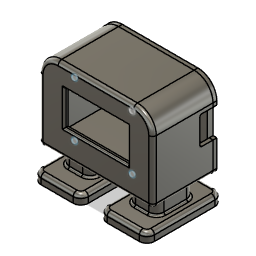
sparky v67 (Autodesk Fusion 360 design; units mm, degrees)
Autodesk Fusion 360 part; units mm, degrees
note: some values were not read from the file. Chosen so that the rebuilt part matches the saved one: which bodies a step acts on; which face or edge a step refers to; which pieces of a blend or face edit are solid.
sketch "Skizze7" plane through (0, 0, 0) normal (0, 1, 0) x (1, 0, 0)
  line L0 (-35, 20) -> (-10, 20)
  line L1 (-10, 20) -> (-10, -20)
  line L2 (-10, -20) -> (-35, -20)
  line L3 (-35, -20) -> (-35, 20)
  line L4 (0, -25) -> (0, 25) construction
  line L5 (35, 20) -> (10, 20)
  line L6 (10, 20) -> (10, -20)
  line L7 (10, -20) -> (35, -20)
  line L8 (35, -20) -> (35, 20)
  dimension "d14" = 25
  dimension "d15" = 40
  constraint horizontal L0
  constraint vertical L1
  constraint horizontal L2
  constraint vertical L3
  constraint parallel L1 L4
  constraint symmetric L0.start L4 L5.start
  constraint symmetric L0.end L4 L5.end
  constraint symmetric L1.end L4 L6.end
  constraint symmetric L2.end L4 L7.end
  measures "d14" distance of L0.start L0.end
  measures "d15" distance of L0.start L2.end
extrude "Extrusion1" add sketch "Skizze7" along normal blind 5 makes body 1 at (-26.6667, 0, -6.6667) makes body 2 at (18.3333, 0, -6.6667)
sketch "Skizze8" plane through (0, 5, 0) normal (0, 1, 0) x (-1, 0, 0)
  line L0 (35, 20) -> (10, 20)
  line L1 (10, 20) -> (10, -20)
  line L2 (10, -20) -> (35, -20)
  line L3 (35, -20) -> (35, 20)
sketch "Skizze9" plane through (0, 5, 0) normal (0, 1, 0) x (-1, 0, 0)
  line L0 (15, -10) -> (27.5, -10)
  line L1 (27.5, -10) -> (27.5, 10)
  line L2 (27.5, 10) -> (15, 10)
  line L3 (15, 10) -> (15, -10)
  line L4 (0, -20) -> (0, 20) construction
  line L5 (-15, -10) -> (-27.5, -10)
  line L6 (-27.5, -10) -> (-27.5, 10)
  line L7 (-27.5, 10) -> (-15, 10)
  line L8 (-15, 10) -> (-15, -10)
  dimension "d18" = 12.5
  dimension "d19" = 20
  constraint horizontal L0
  constraint vertical L1
  constraint horizontal L2
  constraint vertical L3
  constraint perpendicular L0 L4
  constraint symmetric L0.start L4 L5.start
  constraint symmetric L0.end L4 L5.end
  constraint symmetric L1.end L4 L6.end
  constraint symmetric L2.end L4 L7.end
  measures "d18" distance of L0.start L0.end
  measures "d19" distance of L0.start L2.end
extrude "Extrusion2" add sketch "Skizze9" along normal blind 10 bodies 1 2
sketch "Skizze10" plane through (0, 15, 0) normal (0, 1, 0) x (-1, 0, 0)
  line L0 (15, 10) -> (15, -10)
  line L1 (15, -10) -> (27.5, -10)
  line L2 (27.5, -10) -> (27.5, 10)
  line L3 (27.5, 10) -> (15, 10)
  line L4 (-30, -18) -> (30, -18)
  line L5 (30, -18) -> (30, 18)
  line L6 (30, 18) -> (-30, 18)
  line L7 (-30, 18) -> (-30, -18)
  line L8 (-30, -18) -> (30, 18) construction
  line L9 (30, -18) -> (-30, 18) construction
  dimension "d22" = 60
  dimension "d23" = 36
  constraint horizontal L4
  constraint perpendicular L4 L5
  constraint parallel L4 L6
  constraint parallel L5 L7
  constraint coincident L8 origin
  constraint coincident L9 origin
  measures "d22" distance of L5.end L6.end
  measures "d23" distance of L4.end L5.end
extrude "Extrusion3" add sketch "Skizze10" along normal blind 40 contours L0 L1 L2 L3 | L4 L5 L6 L7 bodies 1 2
sketch "Skizze11" plane through (0, 0, -18) normal (0, 0, -1) x (-1, 0, 0)
  line L0 (-30, 15) -> (30, 15)
  line L1 (30, 15) -> (30, 55)
  line L2 (30, 55) -> (-30, 55)
  line L3 (-30, 55) -> (-30, 15)
  line L4 (0, 55) -> (0, 25) construction
  constraint midpoint L2 L4.start
  constraint perpendicular L0 L4
sketch "Skizze12" plane through (0, 0, -18) normal (0, 0, -1) x (1, 0, 0)
ref_plane "Arbeitsebene4" through (0, 35, -14) normal (0, 0, -1) x (-1, 0, 0)
split "Teilen1" by plane through (0, 35, -14) normal (0, 0, -1) bodies 1 makes body 3 at (-26.6667, 5, -18) makes body 4 at (26.6667, 5, -16) makes body 5 at (10, 28.3333, -18)
combine "Kombinieren1" operation add target body 1 tool bodies 3 4
sketch "Skizze13" plane through (0, 0, -14) normal (0, 0, -1) x (-1, 0, 0)
  line L0 (-30, 15) -> (30, 15)
  line L1 (30, 15) -> (30, 55)
  line L2 (30, 55) -> (-30, 55)
  line L3 (-30, 55) -> (-30, 15)
  line L4 (-28, 73) -> (28, 73)
  line L5 (28, 73) -> (28, 17)
  line L6 (28, 17) -> (-28, 17)
  line L7 (-28, 17) -> (-28, 73)
  constraint horizontal L4
  constraint vertical L5
  constraint horizontal L6
  constraint vertical L7
extrude "Extrusion4" cut sketch "Skizze13" against normal blind 30 contours L2 L4 L5 L7 | L2 L5 L6 L7 bodies 1
split "Teilen2" by plane through (0, 15, 0) normal (0, -1, 0) bodies 1 makes body 6 at (26.6667, 0, 6.6667) makes body 7 at (-26.6667, 0, -6.6667)
sketch "Skizze14" plane through (0, 15, 0) normal (0, 1, 0) x (-1, 0, 0)
  line L0 (-15, 10) -> (-27.5, 10)
  line L1 (-27.5, 10) -> (-27.5, -10)
  line L2 (-27.5, -10) -> (-15, -10)
  line L3 (-15, -10) -> (-15, 10)
  circle A0 centre (-21.25, 0.004) radius 2
  line L4 (0, 25) -> (0, -25) construction
  circle A1 centre (21.25, 0.004) radius 2
  dimension "d29" = 4
  constraint vertical L4
  constraint symmetric A0 L4 A1
  measures "d29" diameter of A0
sketch "Skizze16" plane through (0, 55, 0) normal (0, 1, 0) x (-1, 0, 0)
  line L0 (28, 16) -> (28, -14)
  line L1 (28, -14) -> (30, -14)
  line L2 (30, -14) -> (30, 18)
  line L3 (30, 18) -> (-30, 18)
  line L4 (-30, 18) -> (-30, -14)
  line L5 (-30, -14) -> (-28, -14)
  line L6 (-28, -14) -> (-28, 16)
  line L7 (-28, 16) -> (28, 16)
  line L8 (-30, 18) -> (30, 18)
  line L9 (30, 18) -> (30, -14)
  line L10 (30, -14) -> (-30, -14)
  line L11 (-30, -14) -> (-30, 18)
  constraint horizontal L8
  constraint vertical L9
  constraint horizontal L10
  constraint vertical L11
  constraint coincident L1.end L2.start
  constraint coincident L3.end L4.start
extrude "Extrusion6" add sketch "Skizze16" along normal blind 3 contours L0 L1 L2 L3 L4 L5 L6 L7 L8 L9 L10 L11 bodies 1
sketch "Skizze17" plane through (-28, 0, 0) normal (1, 0, 0) x (0, 0, -1)
  line L0 (-16, 58) -> (-16, 17)
  line L1 (-16, 17) -> (14, 17)
  line L2 (14, 17) -> (14, 58)
  line L3 (14, 58) -> (-16, 58)
  line L4 (14, 58) -> (-16, 58)
  line L5 (-16, 58) -> (-16, 56)
  line L6 (-16, 56) -> (14, 56)
  line L7 (14, 56) -> (14, 58)
  constraint horizontal L4
  constraint vertical L5
  constraint horizontal L6
  constraint vertical L7
  constraint coincident L0 L5.end
  constraint coincident L2.end L3.start
extrude "Extrusion7" add sketch "Skizze17" along normal blind 56 contours L0 L2 L3 L4 L5 L6 L7 bodies 1
sketch "Skizze18" plane through (0, 0, 18) normal (0, 0, 1) x (1, 0, 0)
  line L0 (-30, 15) -> (30, 15)
  line L1 (30, 15) -> (30, 58)
  line L2 (30, 58) -> (-30, 58)
  line L3 (-30, 58) -> (-30, 15)
ref_plane "WorkPlane5" through (0, 36.5, 19) normal (0, 0, 1) x (1, 0, 0)
sketch "Sketch19" plane through (0, 0, 19) normal (0, 0, 1) x (1, 0, 0)
  line L0 (-25, 20) -> (25, 20)
  line L1 (25, 20) -> (25, 55)
  line L2 (25, 55) -> (-25, 55)
  line L3 (-25, 55) -> (-25, 20)
  constraint horizontal L0
  constraint vertical L1
  constraint horizontal L2
  constraint vertical L3
sketch "Sketch20" plane through (0, 0, 19) normal (0, 0, 1) x (1, 0, 0)
  line L0 (-17.75, 25) -> (17.75, 25)
  line L1 (17.75, 25) -> (17.75, 48)
  line L2 (17.75, 48) -> (-17.75, 48)
  line L3 (-17.75, 48) -> (-17.75, 25)
  line L4 (-30, 58) -> (-30, 15)
  line L5 (30, 15) -> (30, 58)
  line L6 (30, 58) -> (-30, 58)
  line L7 (-30, 15) -> (30, 15)
  dimension "d37" = 35.5
  dimension "d38" = 23
  dimension "d39" = 12.25
  dimension "d40" = 12.25
  dimension "d41" = 10
  dimension "d42" = 10
  constraint horizontal L0
  constraint vertical L1
  constraint horizontal L2
  constraint vertical L3
  measures "d37" distance of L0.start L0.end
  measures "d38" distance of L0.start L2.end
  measures "d39" distance of L3 L4
  measures "d40" distance of L1 L5
  measures "d41" distance of L2 L6
  measures "d42" distance of L0 L7
extrude "Extrude8" cut sketch "Sketch20" against normal blind 10 contours L0 L1 L2 L3 bodies 1
fillet "Fillet1" radius 8 2 edges at (28, 56, 1) (-28, 56, 1) on bodies 1
fillet "Fillet2" radius 10 2 edges at (-30, 58, 2) (30, 58, 2) on bodies 1
fillet "Fillet3" radius 4 6 edges at (0, 15, 18) (-30, 31.5, 18) (-27.0711, 55.0711, 18) (0, 58, 18) (27.0711, 55.0711, 18) (30, 31.5, 18) on bodies 1
fillet "Fillet4" radius 1 4 edges at (0, 25, 18) (17.75, 36.5, 18) (0, 48, 18) (-17.75, 36.5, 18) on bodies 1
fillet "Fillet5" radius 2 4 edges at (28.8284, 16.1716, 16.8284) (30, 15, 0) (-30, 15, 0) (-28.8284, 16.1716, 16.8284) on bodies 1
fillet "Fillet6" radius 1 2 edges at (-28, 17, 1) (28, 17, 1) on bodies 1
move_body "Move1" bodies 7 to x (1, 0, 0) y (0, 1, 0) z (0, 0, 1) at (-40, 0, 0)
extrude "Extrude9" add 1 faces at (-67.5, 8.3333, -3.3333) along direction (-1, 0, 0) blind 2.5 on bodies 7 bodies 7
delete_body "RemoveBody1" bodies 6
fillet "Fillet7" radius 4 4 edges at (-75, 2.5, 20) (-50, 2.5, 20) (-75, 2.5, -20) (-50, 2.5, -20) on bodies 7
fillet "Fillet8" radius 4 4 edges at (-70, 10, -10) (-70, 10, 10) (-55, 10, -10) (-55, 10, 10) on bodies 7
fillet "Fillet9" radius 2 8 edges at (-73.8284, 5, 18.8284) (-62.5, 5, 20) (-51.1716, 5, 18.8284) (-50, 5, 0) (-51.1716, 5, -18.8284) (-62.5, 5, -20) (-73.8284, 5, -18.8284) (-75, 5, 0) on bodies 7
fillet "Fillet10" radius 1 8 edges at (-56.1716, 5, -8.8284) (-55, 5, 0) (-56.1716, 5, 8.8284) (-62.5, 5, 10) (-68.8284, 5, 8.8284) (-70, 5, 0) (-68.8284, 5, -8.8284) (-62.5, 5, -10) on bodies 7
sketch "Sketch21" plane through (0, 15, 0) normal (0, 1, 0) x (-1, 0, 0)
  arc A0 (59, 10) -> (55, 6) centre (59, 6) ccw
  line L0 (55, 6) -> (55, -6)
  arc A1 (55, -6) -> (59, -10) centre (59, -6) ccw
  line L1 (59, -10) -> (66, -10)
  arc A2 (66, -10) -> (70, -6) centre (66, -6) ccw
  line L2 (70, -6) -> (70, 6)
  arc A3 (70, 6) -> (66, 10) centre (66, 6) ccw
  line L3 (66, 10) -> (59, 10)
  line L4 (57.5, 7.5) -> (67.5, 7.5)
  line L5 (67.5, 7.5) -> (67.5, -7.5)
  line L6 (67.5, -7.5) -> (57.5, -7.5)
  line L7 (57.5, -7.5) -> (57.5, 7.5)
  point P0 (62.5, 0)
  dimension "d67" = 7.5
  dimension "d68" = 10
  constraint horizontal L4
  constraint vertical L5
  constraint horizontal L6
  constraint vertical L7
  measures "d67" distance of L2 P0
  measures "d68" distance of L1 P0
extrude "Extrude10" cut sketch "Sketch21" against normal blind 10 contours L4 L5 L6 L7 bodies 7
fillet "Fillet11" radius 2 1 edges at (-57.5, 10, 7.5) on bodies 7
fillet "Fillet12" radius 2 3 edges at (-67.5, 10, 7.5) (-67.5, 10, -7.5) (-57.5, 10, -7.5) on bodies 7
move_body "Move2" bodies 7 to x (1, 0, 0) y (0, 1, 0) z (0, 0, 1) at (45, 0, 0)
move_body "Move3" bodies 7 to x (1, 0, 0) y (0, 1, 0) z (0, 0, 1) at (0, 0, 1)
copy_body "CopyPasteBodies1" bodies 7 makes body 8
move_body "Move4" bodies 8 to x (1, 0, 0) y (0, 1, 0) z (0, 0, 1) at (35, 0, 0)
sketch "Sketch22" plane through (0, 0, -14) normal (0, 0, -1) x (-1, 0, 0)
  arc A0 (28, 15) -> (30, 17) centre (28, 17) ccw
  line L0 (30, 17) -> (30, 48)
  arc A1 (30, 48) -> (20, 58) centre (20, 48) ccw
  line L1 (20, 58) -> (-20, 58)
  arc A2 (-20, 58) -> (-30, 48) centre (-20, 48) ccw
  line L2 (-30, 48) -> (-30, 17)
  arc A3 (-30, 17) -> (-28, 15) centre (-28, 17) ccw
  line L3 (-28, 15) -> (28, 15)
  arc A4 (27, 17) -> (28, 18) centre (27, 18) ccw
  line L4 (27, 17) -> (-27, 17)
  arc A5 (-28, 18) -> (-27, 17) centre (-27, 18) ccw
  line L5 (-28, 18) -> (-28, 48)
  arc A6 (-20, 56) -> (-28, 48) centre (-20, 48) ccw
  line L6 (-20, 56) -> (20, 56)
  arc A7 (28, 48) -> (20, 56) centre (20, 48) ccw
  line L7 (28, 48) -> (28, 18)
extrude "Extrude11" add sketch "Sketch22" along normal blind 2 separate body makes body 9
delete_body "RemoveBody2" bodies 5
delete_face "DeleteFace1" 1 faces at (27.9989, 17.9524, -14.6667) on bodies 9
delete_face "DeleteFace2" 1 faces at (-27.5, 17.134, -15.3333) on bodies 9
extrude "Extrude12" add 1 faces at (6.6667, 56, -14.6667) along direction (0, -1, 0) blind 40 on bodies 9 bodies 9
extrude "Extrude13" add 1 faces at (22.6667, 17, -14.6667) along direction (0, 1, 0) blind 31 on bodies 9 bodies 9
extrude "Extrude14" add 1 faces at (-25.3333, 17, -14.6667) along direction (0, 1, 0) blind 31 on bodies 9 bodies 9
sketch "Sketch23" plane through (0, 0, -16) normal (0, 0, -1) x (-1, 0, 0)
  arc A0 (-20, 56) -> (-28, 48) centre (-20, 48) ccw
  line L0 (-20, 56) -> (-20, 48)
  line L1 (-20, 48) -> (-28, 48)
  line L2 (-28, 15) -> (28, 15)
  arc A1 (28, 15) -> (30, 17) centre (28, 17) ccw
  line L3 (30, 17) -> (30, 48)
  arc A2 (30, 48) -> (20, 58) centre (20, 48) ccw
  line L4 (20, 58) -> (-20, 58)
  arc A3 (-20, 58) -> (-30, 48) centre (-20, 48) ccw
  line L5 (-30, 48) -> (-30, 17)
  arc A4 (-30, 17) -> (-28, 15) centre (-28, 17) ccw
  line L6 (20, 48) -> (20, 56)
  arc A5 (28, 48) -> (20, 56) centre (20, 48) ccw
  line L7 (28, 48) -> (20, 48)
extrude "Extrude15" add sketch "Sketch23" against normal blind 2 contours A0 L0 L1 bodies 9
sketch "Sketch24" plane through (0, 0, -16) normal (0, 0, -1) x (-1, 0, 0)
  line L0 (-28, 15) -> (28, 15)
  arc A0 (28, 15) -> (30, 17) centre (28, 17) ccw
  line L1 (30, 17) -> (30, 48)
  arc A1 (30, 48) -> (20, 58) centre (20, 48) ccw
  line L2 (20, 58) -> (-20, 58)
  arc A2 (-20, 58) -> (-30, 48) centre (-20, 48) ccw
  line L3 (-30, 48) -> (-30, 17)
  arc A3 (-30, 17) -> (-28, 15) centre (-28, 17) ccw
  line L4 (20, 48) -> (20, 56)
  arc A4 (28, 48) -> (20, 56) centre (20, 48) ccw
  line L5 (28, 48) -> (20, 48)
extrude "Extrude16" add sketch "Sketch24" against normal blind 2 contours L4 A4 L5 bodies 9
delete_face "DeleteFace3" 1 faces at (27.3717, 17.0716, -4) on bodies 1
delete_face "DeleteFace4" 1 faces at (-27.0951, 17.0045, -4) on bodies 1
sketch "Sketch25" plane through (0, 0, 16) normal (0, 0, -1) x (-1, 0, 0)
  line L0 (17.75, 25) -> (-17.75, 25)
  line L1 (-17.75, 25) -> (-17.75, 48)
  line L2 (-17.75, 48) -> (17.75, 48)
  line L3 (17.75, 48) -> (17.75, 25)
  line L4 (28, 17) -> (28, 48)
  arc A0 (28, 48) -> (20, 56) centre (20, 48) ccw
  line L5 (20, 56) -> (-20, 56)
  arc A1 (-20, 56) -> (-28, 48) centre (-20, 48) ccw
  line L6 (-28, 48) -> (-28, 17)
  line L7 (-28, 17) -> (28, 17)
move_body "Move5" bodies 8 7 to x (1, 0, 0) y (0, 1, 0) z (0, 0, 1) at (0, -10, 0)
sketch "Sketch26" plane through (0, 15, 0) normal (0, -1, 0) x (1, 0, 0)
  line L0 (-28, 14) -> (-28, -14)
  line L1 (-28, -14) -> (28, -14)
  line L2 (28, -14) -> (28, 14)
  line L3 (28, 14) -> (-28, 14)
  line L4 (12.5, 6.5) -> (12.5, -4.5)
  arc A0 (12.5, -4.5) -> (14.5, -6.5) centre (14.5, -4.5) ccw
  line L5 (14.5, -6.5) -> (20.5, -6.5)
  arc A1 (20.5, -6.5) -> (22.5, -4.5) centre (20.5, -4.5) ccw
  line L6 (22.5, -4.5) -> (22.5, 6.5)
  arc A2 (22.5, 6.5) -> (20.5, 8.5) centre (20.5, 6.5) ccw
  line L7 (20.5, 8.5) -> (14.5, 8.5)
  arc A3 (14.5, 8.5) -> (12.5, 6.5) centre (14.5, 6.5) ccw
  arc A4 (25, 7) -> (21, 11) centre (21, 7) ccw
  line L8 (25, 7) -> (25, -5)
  arc A5 (21, -9) -> (25, -5) centre (21, -5) ccw
  line L9 (21, -9) -> (14, -9)
  arc A6 (10, -5) -> (14, -9) centre (14, -5) ccw
  line L10 (10, -5) -> (10, 7)
  arc A7 (14, 11) -> (10, 7) centre (14, 7) ccw
  line L11 (14, 11) -> (21, 11)
  line L12 (-22.5, 6.5) -> (-22.5, -4.5)
  arc A8 (-22.5, -4.5) -> (-20.5, -6.5) centre (-20.5, -4.5) ccw
  line L13 (-20.5, -6.5) -> (-14.5, -6.5)
  arc A9 (-14.5, -6.5) -> (-12.5, -4.5) centre (-14.5, -4.5) ccw
  line L14 (-12.5, -4.5) -> (-12.5, 6.5)
  arc A10 (-12.5, 6.5) -> (-14.5, 8.5) centre (-14.5, 6.5) ccw
  line L15 (-14.5, 8.5) -> (-20.5, 8.5)
  arc A11 (-20.5, 8.5) -> (-22.5, 6.5) centre (-20.5, 6.5) ccw
  arc A12 (-10, 7) -> (-14, 11) centre (-14, 7) ccw
  line L16 (-10, 7) -> (-10, -5)
  arc A13 (-14, -9) -> (-10, -5) centre (-14, -5) ccw
  line L17 (-14, -9) -> (-21, -9)
  arc A14 (-25, -5) -> (-21, -9) centre (-21, -5) ccw
  line L18 (-25, -5) -> (-25, 7)
  arc A15 (-21, 11) -> (-25, 7) centre (-21, 7) ccw
  line L19 (-21, 11) -> (-14, 11)
extrude "Extrude17" add sketch "Sketch26" along normal blind 8 contours L4 A0 L5 A1 L6 A2 L7 A3 | L12 A8 L13 A9 L14 A10 L15 A11 bodies 1
delete_face "DeleteFace5" 1 faces at (-13.5, 9.6667, -6.2321) on bodies 1
delete_face "DeleteFace6" 1 faces at (-20.8785, 9.6667, -6.4639) on bodies 1
delete_face "DeleteFace7" 1 faces at (14.1215, 9.6667, -6.4639) on bodies 1
delete_face "DeleteFace8" 1 faces at (20.9715, 9.6667, -6.4436) on bodies 1
delete_face "DeleteFace9" 1 faces at (20.8785, 9.6667, 8.4639) on bodies 1
delete_face "DeleteFace10" 1 faces at (14.4048, 9.6667, 8.4977) on bodies 1
delete_face "DeleteFace11" 1 faces at (-13.1198, 9.6667, 7.9475) on bodies 1
delete_face "DeleteFace12" 1 faces at (-21.9475, 9.6667, 7.8802) on bodies 1
delete_face "DeleteFace13" 1 faces at (-14.4048, 1.6667, -6.4977) on bodies 7
delete_face "DeleteFace14" 1 faces at (-20.9715, 1.6667, -6.4436) on bodies 7
delete_face "DeleteFace15" 1 faces at (-14.4048, 1.6667, 8.4977) on bodies 7
delete_face "DeleteFace16" 1 faces at (-22.4977, 1.6667, 6.5952) on bodies 7
delete_face "DeleteFace17" 1 faces at (12.5023, 1.6667, 6.5952) on bodies 8
delete_face "DeleteFace18" 1 faces at (20.5952, 1.6667, 8.4977) on bodies 8
delete_face "DeleteFace19" 1 faces at (20.5952, 1.6667, -6.4977) on bodies 8
delete_face "DeleteFace20" 1 faces at (13.2637, 1.6667, -6.0721) on bodies 8
sketch "Sketch27" plane through (0, 0, 8.5) normal (0, 0, 1) x (1, 0, 0)
  line L0 (12.5, 7) -> (22.5, 7)
  line L1 (22.5, 7) -> (22.5, 15)
  line L2 (22.5, 15) -> (12.5, 15)
  line L3 (12.5, 15) -> (12.5, 7)
  line L4 (22.5, 15) -> (22.5, 11) construction
  line L5 (22.5, 11) -> (22.5, 8)
  line L6 (22.5, 8) -> (24, 9.5)
  line L7 (24, 9.5) -> (22.5, 11)
  line L8 (22.5, 11) -> (12.5, 11) construction
  line L9 (12.5, 11) -> (12.5, 8)
  line L10 (12.5, 8) -> (11, 9.5)
  line L11 (11, 9.5) -> (12.5, 11)
  constraint coincident L1.end L2.start
  constraint midpoint L1 L4.end
  constraint coincident L1 L5.end
  constraint parallel L1 L5
  constraint perpendicular L1 L8
  constraint coincident L3 L9.end
sketch "Sketch28" plane through (0, 0, 8.5) normal (0, 0, 1) x (1, 0, 0)
  line L0 (-22.5, 7) -> (-12.5, 7)
  line L1 (-12.5, 7) -> (-12.5, 15)
  line L2 (-12.5, 15) -> (-22.5, 15)
  line L3 (-22.5, 15) -> (-22.5, 7)
  line L4 (-12.5, 15) -> (-12.5, 11) construction
  line L5 (-12.5, 11) -> (-12.5, 8)
  line L6 (-12.5, 8) -> (-11, 9.5)
  line L7 (-11, 9.5) -> (-12.5, 11)
  line L8 (-22.5, 8) -> (-22.5, 11)
  line L9 (-22.5, 11) -> (-24, 9.5)
  line L10 (-24, 9.5) -> (-22.5, 8)
  constraint coincident L1.end L2.start
  constraint midpoint L1 L4.end
  constraint coincident L1 L5.end
  constraint perpendicular L0 L5
  constraint coincident L3 L8.start
  constraint midpoint L3 L8.end
  constraint perpendicular L7 L9
extrude "Extrude18" add sketch "Sketch27" sketch "Sketch28" against normal blind 15 contours L3 L9 L10 L11 | L1 L5 L6 L7 of sketch 2 contours L3 L8 L9 L10 | L1 L5 L6 L7 bodies 1
sketch "Sketch29" plane through (0, 0, -6.5) normal (0, 0, -1) x (-1, 0, 0)
  line L0 (22.5, 7) -> (22.5, 8)
  line L1 (22.5, 8) -> (24, 9.5)
  line L2 (24, 9.5) -> (22.5, 11)
  line L3 (22.5, 11) -> (22.5, 15)
  line L4 (22.5, 15) -> (12.5, 15)
  line L5 (12.5, 15) -> (12.5, 11)
  line L6 (12.5, 11) -> (11, 9.5)
  line L7 (11, 9.5) -> (12.5, 8)
  line L8 (12.5, 8) -> (12.5, 7)
  line L9 (12.5, 7) -> (22.5, 7)
  line L10 (21.5, 7) -> (13.5, 7)
  line L11 (13.5, 7) -> (13.5, 15)
  line L12 (13.5, 15) -> (21.5, 15)
  line L13 (21.5, 15) -> (21.5, 7)
  line L14 (-13.5, 7) -> (-21.5, 7)
  line L15 (-21.5, 7) -> (-21.5, 15)
  line L16 (-21.5, 15) -> (-13.5, 15)
  line L17 (-13.5, 15) -> (-13.5, 7)
  constraint horizontal L10
  constraint vertical L11
  constraint horizontal L12
  constraint vertical L13
  constraint coincident L4 L11.end
  constraint coincident L9 L10.start
  constraint horizontal L14
  constraint vertical L15
  constraint horizontal L16
  constraint vertical L17
extrude "Extrude19" cut sketch "Sketch29" against normal blind 47 contours L4 L9 L10 L11 L12 L13 | L14 L15 L16 L17 bodies 1
ref_plane "WorkPlane6" through (24, 7.5, 1) normal (1, 0, 0) x (0, 0, 1)
sketch "Sketch30" plane through (24, 0, 0) normal (1, 0, 0) x (0, 0, -1)
  line L0 (-8.5, 15) -> (-1.5, 8)
  line L1 (-14, 15) -> (14, 15)
  line L2 (-1.5, 8) -> (-0.5, 7)
  line L3 (-0.5, 7) -> (-8.5, 7)
  line L4 (-8.5, 7) -> (-8.5, 15)
  dimension "d94" = 7
  dimension "d95" = 45
  constraint parallel L0 L2
  constraint horizontal L3
  constraint coincident L0.start L4.end
  measures "d94" horizontal distance of L0.start L0.end
  measures "d95" angle of L0 L1
extrude "Extrude20" cut sketch "Sketch30" against normal blind 97 bodies 1
extrude "Extrude21" add 1 faces at (21.5, 12.6667, 1.1667) along direction (-1, 0, 0) blind 0.5 on bodies 1 bodies 1
extrude "Extrude22" add 1 faces at (13.5, 12.6667, 1.1667) along direction (1, 0, 0) blind 0.5 on bodies 1 bodies 1
extrude "Extrude23" add 1 faces at (-13.5, 12.6667, 1.1667) along direction (-1, 0, 0) blind 0.5 on bodies 1 bodies 1
extrude "Extrude24" add 1 faces at (-21.5, 12.6667, 1.1667) along direction (1, 0, 0) blind 0.5 on bodies 1 bodies 1
delete_face "DeleteFace21" 1 faces at (-6.1868, 24.0636, 17.998) on bodies 1
delete_face "DeleteFace22" 1 faces at (-18.4678, 40.8126, 17.9594) on bodies 1
delete_face "DeleteFace23" 1 faces at (6.3959, 48.7178, 17.9594) on bodies 1
delete_face "DeleteFace24" 1 faces at (18.7024, 40.3333, 17.9989) on bodies 1
extrude "Extrude25" add 1 faces at (5.9167, 25, 16.6667) along direction (0, 1, 0) blind 3 on bodies 1 bodies 1
fillet "Fillet13" radius 1 4 edges at (0, 28, 18) (-17.75, 38, 18) (0, 48, 18) (17.75, 38, 18) on bodies 1
sketch "Sketch31" plane through (0, 0, 16) normal (0, 0, -1) x (-1, 0, 0)
  circle A0 centre (-12.6, 50.9) radius 2.5
  circle A1 centre (12.8, 50.9) radius 2.5
  circle A2 centre (-12.6, 23.2) radius 2.5
  circle A3 centre (12.8, 23.2) radius 2.5
  dimension "d110" = 5
  dimension "d111" = 5
  dimension "d112" = 25.4
  dimension "d113" = 5
  dimension "d114" = 27.7
  dimension "d115" = 5
  dimension "d116" = 25.4
  measures "d110" diameter of A0
  measures "d111" diameter of A1
  measures "d112" distance of A0.centre A1.centre
  measures "d113" diameter of A2
  measures "d114" distance of A0.centre A2.centre
  measures "d115" diameter of A3
  measures "d116" distance of A2.centre A3.centre
extrude "Extrude26" add sketch "Sketch31" along normal blind 3 bodies 1
sketch "Sketch32" plane through (0, 0, 0) normal (0, 0, 1) x (1, 0, 0)
  circle A0 centre (12.6, 50.9) radius 1.5
  circle A1 centre (-12.8, 50.9) radius 1.5
  circle A2 centre (12.6, 23.2) radius 1.5
  circle A3 centre (-12.8, 23.2) radius 1.5
  point P0 (12.6, 50.9)
  dimension "d119" = 3
  dimension "d120" = 3
  dimension "d121" = 3
  dimension "d122" = 3
  constraint coincident P0 A0.centre
  measures "d119" diameter of A0
  measures "d120" diameter of A1
  measures "d121" diameter of A2
  measures "d122" diameter of A3
extrude "Extrude27" add sketch "Sketch32" against normal blind 4 separate body makes body 10 at (-14.1822, 50.3173, -2.6667) makes body 11 at (-11.3019, 23.1252, -2.6667) makes body 12 at (14.0095, 50.387, -2.6667) makes body 13 at (14.0981, 23.1252, -2.6667)
move_body "Move6" bodies 10 11 12 13 to x (1, 0, 0) y (0, 1, 0) z (0, 0, 1) at (0, 0, 13)
extrude "Extrude28" add 4 faces at (-12.4753, 51.333, 9) (-12.3495, 22.9831, 9) (12.4887, 51.3875, 9) (13.0505, 22.9831, 9) along direction (0, 0, -1) blind 1 on bodies 10 11 12 13 bodies 10 11 12 13
fillet "Fillet14" radius 0.5 4 edges at (-14.1985, 51.4424, 8) (-14.1985, 23.7424, 8) (11.2015, 51.4424, 8) (11.2015, 23.7424, 8) on bodies 10 11 12 13
combine "Combine2" operation add target body 1 tool bodies 10 11 12 13
move_body "Move7" bodies 9 to x (1, 0, 0) y (0, 1, 0) z (0, 0, 1) at (0, 0, -15)
sketch "Sketch33" plane through (0, 0, -29) normal (0, 0, 1) x (1, 0, 0)
  line L0 (-28, 15) -> (28, 15)
  arc A0 (28, 15) -> (30, 17) centre (28, 17) ccw
  line L1 (30, 17) -> (30, 48)
  arc A1 (30, 48) -> (20, 58) centre (20, 48) ccw
  line L2 (20, 58) -> (-20, 58)
  arc A2 (-20, 58) -> (-30, 48) centre (-20, 48) ccw
  line L3 (-30, 48) -> (-30, 17)
  arc A3 (-30, 17) -> (-28, 15) centre (-28, 17) ccw
  line L4 (-28, 48) -> (-28, 17)
  line L5 (-28, 17) -> (28, 17)
  line L6 (28, 17) -> (28, 48)
  arc A4 (28, 48) -> (20, 56) centre (20, 48) ccw
  line L7 (20, 56) -> (-20, 56)
  arc A5 (-20, 56) -> (-28, 48) centre (-20, 48) ccw
  arc A6 (-30, 17) -> (-28, 15) centre (-28, 17) ccw
  line L8 (-30, 17) -> (-30, 48)
  arc A7 (-20, 58) -> (-30, 48) centre (-20, 48) ccw
  line L9 (-20, 58) -> (20, 58)
  arc A8 (30, 48) -> (20, 58) centre (20, 48) ccw
  line L10 (30, 48) -> (30, 17)
  arc A9 (28, 15) -> (30, 17) centre (28, 17) ccw
  line L11 (28, 15) -> (-28, 15)
extrude "Extrude29" add sketch "Sketch33" along normal blind 2 contours L4 L5 L6 A4 L7 A5 bodies 9
extrude "Extrude30" cut 1 faces at (6.6667, 30, -27) along direction (0, 0, -1) blind 1 on bodies 9 bodies 9
sketch "Sketch34" plane through (0, 0, -28) normal (0, 0, 1) x (1, 0, 0)
  arc A0 (-20, 56) -> (-28, 48) centre (-20, 48) ccw
  line L0 (-28, 48) -> (-28, 17)
  line L1 (-28, 17) -> (28, 17)
  line L2 (28, 17) -> (28, 48)
  arc A1 (28, 48) -> (20, 56) centre (20, 48) ccw
  line L3 (20, 56) -> (-20, 56)
  circle A2 centre (-23.5, 49.5) radius 1.5
  circle A3 centre (23.5, 49.5) radius 1.5
  circle A4 centre (-23.5, 26.5) radius 1.5
  circle A5 centre (23.5, 26.5) radius 1.5
  dimension "d134" = 3
  dimension "d135" = 3
  dimension "d136" = 47
  dimension "d137" = 4.5
  dimension "d138" = 6.5
  dimension "d139" = 6.5
  dimension "d140" = 3
  dimension "d141" = 23
  dimension "d142" = 3
  dimension "d143" = 47
  dimension "d144" = 23
  measures "d134" diameter of A2
  measures "d135" diameter of A3
  measures "d136" horizontal distance of A2.centre A3.centre
  measures "d137" distance of L0 A2.centre
  measures "d138" distance of L3 A2.centre
  measures "d139" distance of L3 A3.centre
  measures "d140" diameter of A4
  measures "d141" distance of A2.centre A4.centre
  measures "d142" diameter of A5
  measures "d143" distance of A4.centre A5.centre
  measures "d144" distance of A3.centre A5.centre
extrude "Extrude31" cut sketch "Sketch34" against normal up to surface (3 mm away) contours A2 | A3 | A4 | A5 bodies 9
sketch "Sketch35" plane through (-30, 0, 0) normal (-1, 0, 0) x (0, 0, 1)
  line L0 (-14, 17) -> (14, 17)
  line L1 (14, 17) -> (14, 48)
  line L2 (14, 48) -> (-14, 48)
  line L3 (-14, 48) -> (-14, 17)
  line L4 (-14, 43) -> (-7, 43)
  line L5 (-7, 43) -> (-7, 31)
  line L6 (-7, 31) -> (-14, 31)
  line L7 (-14, 31) -> (-14, 43)
  constraint horizontal L4
  constraint vertical L5
  constraint horizontal L6
  constraint vertical L7
  constraint coincident L3 L4.start
extrude "Extrude32" cut sketch "Sketch35" against normal up to surface (2 mm away) contours L3 L4 L5 L6 L7 bodies 1
fillet "Fillet15" radius 1 2 edges at (-29, 43, -7) (-29, 31, -7) on bodies 1
sketch "Sketch36" plane through (28, 0, 0) normal (-1, 0, 0) x (0, 0, 1)
  line L0 (-14, 17) -> (16, 17)
  line L1 (16, 17) -> (16, 48)
  line L2 (16, 48) -> (-14, 48)
  line L3 (-14, 48) -> (-14, 17)
  line L4 (-14, 31) -> (-8, 31)
  arc A0 (-8, 31) -> (-7, 32) centre (-8, 32) ccw
  line L5 (-7, 32) -> (-7, 42)
  arc A1 (-7, 42) -> (-8, 43) centre (-8, 42) ccw
  line L6 (-8, 43) -> (-14, 43)
extrude "Extrude33" cut sketch "Sketch36" against normal up to surface (2 mm away) contours L3 L4 A0 L5 A1 L6 bodies 1
sketch "Sketch37" plane through (0, 0, 0) normal (1, 0, 0) x (0, 0, -1)
  line L0 (28, 56) -> (18, 56)
  line L1 (18, 56) -> (18, 54)
  line L2 (18, 54) -> (28, 54)
  line L3 (28, 54) -> (28, 56)
  line L4 (28, 17) -> (18, 17)
  line L5 (18, 17) -> (18, 19)
  line L6 (18, 19) -> (28, 19)
  line L7 (28, 19) -> (28, 17)
  line L8 (20, 56) -> (21.5, 57.5)
  line L9 (20, 56) -> (22.1213, 56) construction
  line L10 (21.5, 57.5) -> (23, 56)
  line L11 (20, 54) -> (23, 54)
  line L12 (20, 17) -> (23, 17)
  line L13 (23, 17) -> (21.5, 15.5)
  line L14 (21.5, 15.5) -> (20, 17)
  dimension "d153" = 10
  dimension "d154" = 2
  dimension "d155" = 10
  dimension "d156" = 2
  dimension "d157" = 45
  constraint horizontal L0
  constraint vertical L1
  constraint horizontal L2
  constraint vertical L3
  constraint horizontal L4
  constraint vertical L5
  constraint horizontal L6
  constraint vertical L7
  constraint horizontal L9
  constraint coincident L0 L8.start
  constraint midpoint L0 L10.end
  constraint coincident L2 L11.start
  constraint midpoint L2 L11.end
  constraint coincident L4 L12.start
  constraint midpoint L4 L12.end
  measures "d153" distance of L0.start L0.end
  measures "d154" distance of L0.start L2.end
  measures "d155" distance of L4.start L4.end
  measures "d156" distance of L4.start L6.end
  measures "d157" angle of L8 L9
extrude "Extrude34" add sketch "Sketch37" along normal mid plane 8 bodies 9
move_body "Move8" bodies 9 to x (1, 0, 0) y (0, 1, 0) z (0, 0, 1) at (0, 0, 15)
sketch "Sketch38" plane through (4, 0, 0) normal (1, 0, 0) x (0, 0, -1)
  line L0 (6.5, 15.5) -> (8, 17)
  line L1 (8, 17) -> (13, 17)
  line L2 (13, 17) -> (13, 19)
  line L3 (13, 19) -> (3, 19)
  line L4 (3, 19) -> (3, 17)
  line L5 (3, 17) -> (5, 17)
  line L6 (5, 17) -> (6.5, 15.5)
  line L7 (5, 17) -> (8, 17)
  line L8 (6.5, 15.5) -> (8, 17)
  line L9 (6.5, 15.5) -> (5, 17)
  line L10 (5, 56) -> (8, 56)
  line L11 (8, 56) -> (6.5, 57.5)
  line L12 (6.5, 57.5) -> (5, 56)
  constraint coincident L5.end L6.start
  constraint coincident L0.end L1.start
  constraint coincident L0.start L6.end
  constraint parallel L3 L10
  constraint parallel L6 L11
extrude "Extrude35" cut sketch "Sketch38" against normal blind 8 contours L0 L6 L7 L8 L9 | L10 L11 L12 bodies 1
move_body "Move9" bodies 9 to x (1, 0, 0) y (0, 1, 0) z (0, 0, 1) at (0, 0, -16)
move_body "Move10" bodies 8 7 to x (1, 0, 0) y (0, 1, 0) z (0, 0, 1) at (0, 10, 0)
sketch "Sketch39" plane through (0, 3.25, -3.25) normal (0, -0.707107, 0.707107) x (1, 0, 0)
  line L0 (-14, 6.7175) -> (-12.5, 6.7175)
  line L1 (-12.5, 6.7175) -> (-11, 8.8388)
  line L2 (-11, 8.8388) -> (-12.5, 10.9602)
  line L3 (-12.5, 10.9602) -> (-12.5, 16.617)
  line L4 (-12.5, 16.617) -> (-14, 16.617)
  line L5 (-14, 16.617) -> (-14, 6.7175)
sketch "Sketch40" plane through (0, 0, -6.5) normal (0, 0, -1) x (-1, 0, 0)
  line L0 (-21, 15) -> (-22.5, 15)
  line L1 (-22.5, 15) -> (-22.5, 11)
  line L2 (-22.5, 11) -> (-24, 9.5)
  line L3 (-24, 9.5) -> (-22.5, 8)
  line L4 (-22.5, 8) -> (-22.5, 7)
  line L5 (-22.5, 7) -> (-21, 7)
  line L6 (-21, 7) -> (-21, 15)
  line L7 (-24, 9.5) -> (-22.5, 11)
  line L8 (-22.5, 8) -> (-22.5, 11)
  line L9 (-24, 9.5) -> (-22.5, 8)
  line L10 (-12.5, 8) -> (-12.5, 11)
  line L11 (-12.5, 11) -> (-11, 9.5)
  line L12 (-11, 9.5) -> (-12.5, 8)
  line L13 (12.5, 11) -> (11, 9.5)
  line L14 (11, 9.5) -> (12.5, 8)
  line L15 (12.5, 8) -> (12.5, 11)
  line L16 (22.5, 11) -> (22.5, 8)
  line L17 (22.5, 8) -> (24, 9.5)
  line L18 (24, 9.5) -> (22.5, 11)
  constraint coincident L2.end L3.start
  constraint coincident L1.end L2.start
  constraint coincident L3.end L4.start
  constraint parallel L4 L10
  constraint parallel L3 L11
  constraint perpendicular L11 L13
  constraint perpendicular L13 L14
  constraint vertical L15
  constraint parallel L15 L16
  constraint parallel L13 L17
extrude "Extrude36" cut sketch "Sketch40" against normal blind 15 contours L2 L3 L7 L8 L9 | L10 L11 L12 | L13 L14 L15 | L16 L17 L18 bodies 7 8
move_body "Move11" bodies 7 8 to x (1, 0, 0) y (0, 1, 0) z (0, 0, 1) at (0, -14, 0)
move_body "Move12" bodies 1 7 8 9 to x (1, 0, 0) y (0, 1, 0) z (0, 0, 1) at (0, 14, 0)
move_body "Move13" bodies 1 to x (1, 0, 0) y (0, 1, 0) z (0, 0, 1) at (0, -14, 0)
move_body "Move14" bodies 9 to x (1, 0, 0) y (0, 1, 0) z (0, 0, 1) at (0, -14, 0)
move_body "Move15" bodies 9 to x (1, 0, 0) y (0, 1, 0) z (0, 0, 1) at (0, 0, 16)
delete_face "DeleteFace25" 1 faces at (11.1551, 50.5321, 8.4054) on bodies 1
delete_face "DeleteFace26" 1 faces at (-13.2038, 49.4648, 8.4054) on bodies 1
delete_face "DeleteFace27" 1 faces at (-14.2836, 23.0515, 8.4054) on bodies 1
delete_face "DeleteFace28" 1 faces at (11.9868, 21.841, 8.4054) on bodies 1
delete_face "DeleteFace29" 2 faces at (11.3201, 50.1178, 9.6667) (13.627, 50.6273, 8) on bodies 1
delete_face "DeleteFace30" 1 faces at (10.2963, 51.8711, 14) on bodies 1
delete_face "DeleteFace31" 2 faces at (-14.2095, 50.387, 9.6667) (-13.1247, 50.467, 8) on bodies 1
delete_face "DeleteFace32" 1 faces at (-15.2969, 50.7754, 14) on bodies 1
delete_face "DeleteFace33" 2 faces at (-11.3019, 23.1252, 9.6667) (-13.27, 22.7338, 8) on bodies 1
delete_face "DeleteFace34" 1 faces at (-15.2876, 22.9511, 15) on bodies 1
delete_face "DeleteFace35" 2 faces at (14.0981, 23.1252, 9.6667) (12.9865, 23.5909, 8) on bodies 1
delete_face "DeleteFace36" 1 faces at (10.1124, 22.9511, 15) on bodies 1
delete_face "DeleteFace37" 1 faces at (18.6864, 34.3966, 17.998) on bodies 1
delete_face "DeleteFace38" 1 faces at (-6.3959, 48.7178, 17.9594) on bodies 1
delete_face "DeleteFace39" 1 faces at (-6.3959, 27.2822, 17.9594) on bodies 1
delete_face "DeleteFace40" 1 faces at (-17.8612, 34.6667, 17.4582) on bodies 1
sketch "Sketch41" plane through (0, 0, 16) normal (0, 0, -1) x (-1, 0, 0)
  line L0 (17.75, 28) -> (-17.75, 28)
  line L1 (-17.75, 28) -> (-17.75, 48)
  line L2 (-17.75, 48) -> (17.75, 48)
  line L3 (17.75, 48) -> (17.75, 28)
  line L4 (28, 17) -> (28, 48)
  arc A0 (28, 48) -> (20, 56) centre (20, 48) ccw
  line L5 (20, 56) -> (-20, 56)
  arc A1 (-20, 56) -> (-28, 48) centre (-20, 48) ccw
  line L6 (-28, 48) -> (-28, 17)
  line L7 (-28, 17) -> (28, 17)
  circle A2 centre (-15.25, 51) radius 2.5
  circle A3 centre (15.25, 51) radius 2.5
  circle A4 centre (-15.25, 22) radius 2.5
  circle A5 centre (15.25, 22) radius 2.5
  dimension "d164" = 5
  dimension "d165" = 5
  dimension "d166" = 5
  dimension "d167" = 5
  dimension "d173" = 12.75
  dimension "d174" = 12.75
  dimension "d175" = 30.5
  dimension "d176" = 5
  dimension "d177" = 5
  dimension "d178" = 12.75
  dimension "d179" = 12.75
  dimension "d180" = 5
  dimension "d181" = 5
  dimension "d182" = 29
  dimension "d183" = 29
  measures "d164" diameter of A2
  measures "d165" diameter of A3
  measures "d166" diameter of A4
  measures "d167" diameter of A5
  measures "d173" distance of L6 A2.centre
  measures "d174" distance of L4 A3.centre
  measures "d175" horizontal distance of A2.centre A3.centre
  measures "d176" distance of L5 A2.centre
  measures "d177" distance of L5 A3.centre
  measures "d178" distance of L6 A4.centre
  measures "d179" distance of L4 A5.centre
  measures "d180" distance of L7 A4.centre
  measures "d181" distance of L7 A5.centre
  measures "d182" distance of A2.centre A4.centre
  measures "d183" distance of A3.centre A5.centre
extrude "Extrude37" add sketch "Sketch41" along normal blind 2 contours A2 | A3 | A4 | A5 bodies 1
extrude "Extrude38" add 1 faces at (-5.9167, 28, 16.6667) along direction (0, 1, 0) blind 1 on bodies 1 bodies 1
extrude "Extrude39" add 1 faces at (17.75, 35.3333, 16.6667) along direction (-1, 0, 0) blind 1 on bodies 1 bodies 1
extrude "Extrude40" add 1 faces at (-17.75, 41.6667, 16.6667) along direction (1, 0, 0) blind 1 on bodies 1 bodies 1
extrude "Extrude41" add 1 faces at (5.5833, 48, 17.3333) along direction (0, -1, 0) blind 1 on bodies 1 bodies 1
fillet "Fillet16" radius 1 4 edges at (0, 47, 18) (16.75, 38, 18) (0, 29, 18) (-16.75, 38, 18) on bodies 1
sketch "Sketch42" plane through (0, 0, 14) normal (0, 0, -1) x (-1, 0, 0)
  circle A0 centre (-15.25, 51) radius 2.5
  circle A1 centre (-15.25, 51) radius 1.45
  circle A2 centre (15.25, 51) radius 1.45
  circle A3 centre (15.25, 22) radius 1.45
  circle A4 centre (-15.25, 22) radius 1.45
  dimension "d196" = 2.9
  dimension "d197" = 2.9
  dimension "d198" = 2.9
  dimension "d199" = 2.9
  constraint concentric A0 A1
  measures "d196" diameter of A1
  measures "d197" diameter of A2
  measures "d198" diameter of A3
  measures "d199" diameter of A4
extrude "Extrude42" cut sketch "Sketch42" against normal blind 2 contours A1 | A2 | A3 | A4 bodies 1
delete_face "DeleteFace41" 1 faces at (29.3333, 42.5, -7.134) on bodies 1
delete_face "DeleteFace42" 1 faces at (-29.3333, 42.7237, -7.3099) on bodies 1
extrude "Extrude43" cut 2 faces at (-29.3333, 43, -11.6667) (28.6667, 43, -9.3333) along direction (0, 1, 0) blind 3 on bodies 1 bodies 1
fillet "Fillet17" radius 1 2 edges at (-29, 46, -7) (29, 46, -7) on bodies 1
delete_face "DeleteFace43" 1 faces at (-1.3333, 16, -6) on bodies 9
delete_face "DeleteFace44" 1 faces at (1.3333, 57, -6) on bodies 9
extrude "Extrude44" cut 1 faces at (1.3333, 54.6667, -3) along direction (0, 0, -1) blind 10 on bodies 9 bodies 9
extrude "Extrude45" cut 1 faces at (-1.3333, 17.6667, -3) along direction (0, 0, -1) blind 10 on bodies 9 bodies 9
delete_face "DeleteFace45" 1 faces at (1.3333, 16, -7) on bodies 1
delete_face "DeleteFace46" 1 faces at (1.3333, 56.5, -7.5) on bodies 1
split "Split3" by plane through (0, 15, 0) normal (0, -1, 0) bodies 1 makes body 14 at (21, 12.6667, 1.1667) makes body 15 at (-21, 12.6667, 1.1667) makes body 16 at (-14, 12.6667, 1.1667) makes body 17 at (14, 12.6667, 1.1667)
move_body "Move16" bodies 14 to x (1, 0, 0) y (0, 1, 0) z (0, 0, 1) at (-0.5, 0, 0)
move_body "Move17" bodies 17 to x (1, 0, 0) y (0, 1, 0) z (0, 0, 1) at (0.5, 0, 0)
move_body "Move18" bodies 16 to x (1, 0, 0) y (0, 1, 0) z (0, 0, 1) at (-0.5, 0, 0)
move_body "Move19" bodies 15 to x (1, 0, 0) y (0, 1, 0) z (0, 0, 1) at (0.5, 0, 0)
combine "Combine3" operation add target body 1 tool bodies 14 15 16 17
extrude "Extrude46" add 4 faces at (-17.2326, 22.8169, 14) (17.2326, 22.8169, 14) (-16.6818, 52.5962, 14) (13.1147, 50.8038, 14) along direction (0, 0, -1) blind 1 on bodies 1 bodies 1
sketch "Sketch43" plane through (0, 0, -14) normal (0, 0, 1) x (1, 0, 0)
  line L0 (-20, 56) -> (20, 56)
  arc A0 (28, 48) -> (20, 56) centre (20, 48) ccw
  line L1 (28, 48) -> (28, 17)
  line L2 (28, 17) -> (-28, 17)
  line L3 (-28, 17) -> (-28, 48)
  arc A1 (-20, 56) -> (-28, 48) centre (-20, 48) ccw
  line L4 (-28, 15) -> (28, 15)
  arc A2 (28, 15) -> (30, 17) centre (28, 17) ccw
  line L5 (30, 17) -> (30, 48)
  arc A3 (30, 48) -> (20, 58) centre (20, 48) ccw
  line L6 (20, 58) -> (-20, 58)
  arc A4 (-20, 58) -> (-30, 48) centre (-20, 48) ccw
  line L7 (-30, 48) -> (-30, 17)
  arc A5 (-30, 17) -> (-28, 15) centre (-28, 17) ccw
  line L8 (28, 46) -> (30, 46)
  line L9 (30, 46) -> (30, 31)
  line L10 (30, 31) -> (28, 31)
  line L11 (28, 31) -> (28, 46)
  line L12 (-28, 46) -> (-30, 46)
  line L13 (-30, 46) -> (-30, 31)
  line L14 (-30, 31) -> (-28, 31)
  line L15 (-28, 31) -> (-28, 46)
  constraint coincident L1 L8.start
  constraint coincident L5 L8.end
  constraint perpendicular L5 L8
  constraint coincident L5 L9.end
  constraint perpendicular L8 L9
  constraint coincident L1 L10.end
  constraint perpendicular L1 L10
  constraint coincident L3 L12.start
  constraint coincident L7 L12.end
  constraint perpendicular L7 L12
  constraint coincident L7 L13.end
  constraint coincident L3 L14.end
  constraint perpendicular L3 L14
extrude "Extrude47" cut sketch "Sketch43" against normal blind 2 contours L3 L7 L12 L13 L14 L15 | L1 L5 L8 L9 L10 L11 bodies 9
delete_face "DeleteFace47" 8 faces at (29.6479, 50.3405, 14.757) (6.6667, 57.1442, 16.4726) (-29.8828, 48.9437, 14.757) (-29.0572, 27.6447, 16.5795) (-27.5938, 16.4841, 17.0825) (-9.1463, 15.8641, 16.4831) (27.5938, 16.4841, 17.0825) (29.0572, 27.6447, 16.5795) on bodies 1
fillet "Fillet18" radius 2 8 edges at (30, 32.5, 18) (29.4142, 15.5858, 18) (0, 15, 18) (-29.4142, 15.5858, 18) (-30, 32.5, 18) (-27.0711, 55.0711, 18) (0, 58, 18) (27.0711, 55.0711, 18) on bodies 1
extrude "Extrusion5" [suppressed]
sketch "Skizze15" plane through (0, 17, 0) normal (0, 1, 0) x (-1, 0, 0)
  line L0 (-28, -14) -> (28, -14)
  line L1 (28, -14) -> (28, 16)
  line L2 (28, 16) -> (-28, 16)
  line L3 (-28, 16) -> (-28, -14)
sketch "Skizze1" plane through (0, 0, 0) normal (0, 1, 0) x (1, 0, 0)
  line L0 (0, 0) -> (55, 0) construction
  line L1 (55, 0) -> (55, -70) construction
  line L2 (55, -70) -> (0, -70) construction
  line L3 (0, -70) -> (0, 0) construction
  circle A0 centre (27.5, -35) radius 50
  point P0 (77.5, -35)
  dimension "d1" = 55
  dimension "d2" = 70
  dimension "d3" = 100
  constraint horizontal L0
  constraint vertical L1
  constraint horizontal L2
  constraint vertical L3
  constraint coincident L0.start L3.end
  constraint coincident A0 P0
  measures "d1" distance of L0.start L0.end
  measures "d2" distance of L0.start L2.end
  measures "d3" diameter of A0
ref_plane "Arbeitsebene1" through (0, 0, 35) normal (0, 0, 1) x (1, 0, 0)
sketch "Skizze2" plane through (0, 0, 35) normal (0, 0, 1) x (1, 0, 0)
  line L0 (27.5, 0) -> (77.5, 0)
  line L1 (27.5, 0) -> (27.5, 70)
  line L2 (27.5, 0) -> (73.3861, 65.5322) construction
  line L3 (27.5, 0) -> (97.5, 0) construction
  line L4 (77.5, 0) -> (73.3861, 65.5322) construction
  line L5 (73.3861, 65.5322) -> (60, 70) construction
  line L6 (60, 70) -> (27.5, 70) construction
  spline S0 degree 3 poles (77.5, 0) (73.3861, 65.5322) (60, 70) (27.5, 70) knots 0 0 0 0 1 1 1 1
  dimension "d5" = 70
  dimension "d6" = 80
  dimension "d7" = 55
  constraint horizontal L0
  constraint perpendicular L0 L1
  constraint horizontal L3
  measures "d5" distance of L0.start L1.end
  measures "d6" distance of L0.start L2.end
  measures "d7" angle of L2 L3
revolve "Drehen1" [suppressed]
sketch "Skizze3" plane through (0, 0, 0) normal (0, 1, 0) x (1, 0, 0)
  point P0 (27.5, -35)
  point P1 (27.5, -85)
ref_plane "Arbeitsebene2" through (0, 0, 85) normal (0, 0, 1) x (1, 0, 0)
sketch "Skizze5" plane through (0, 0, 0) normal (0, 1, 0) x (1, 0, 0)
  line L0 (27.5, -85) -> (27.5, -70) construction
  constraint vertical L0
ref_plane "Arbeitsebene3" through (0, 0, 70) normal (0, 0, 1) x (1, 0, 0)
sketch "Skizze6" plane through (0, 0, 70) normal (0, 0, 1) x (1, 0, 0)
  line L0 (27.5, 0) -> (27.5, 20) construction
  line L1 (10, 32.5) -> (45, 32.5)
  line L2 (45, 32.5) -> (45, 7.5)
  line L3 (45, 7.5) -> (10, 7.5)
  line L4 (10, 7.5) -> (10, 32.5)
  line L5 (10, 32.5) -> (45, 7.5) construction
  line L6 (45, 32.5) -> (10, 7.5) construction
  point P0 (27.5, 20)
  dimension "d11" = 20
  dimension "d12" = 35
  dimension "d13" = 25
  constraint vertical L0
  constraint horizontal L1
  constraint perpendicular L1 L2
  constraint parallel L1 L3
  constraint parallel L2 L4
  constraint coincident L5 P0
  constraint coincident L6 P0
  constraint coincident P0 L0.end
  measures "d11" distance of L0.start P0
  measures "d12" distance of L2.end L3.end
  measures "d13" distance of L1.end L2.end
named bodies: "Body", "Back Lid", "Left Feet", "Feet", "Feet (1)", "Body (1)", "Body (2)", "Body (3)", "Body (4)"
